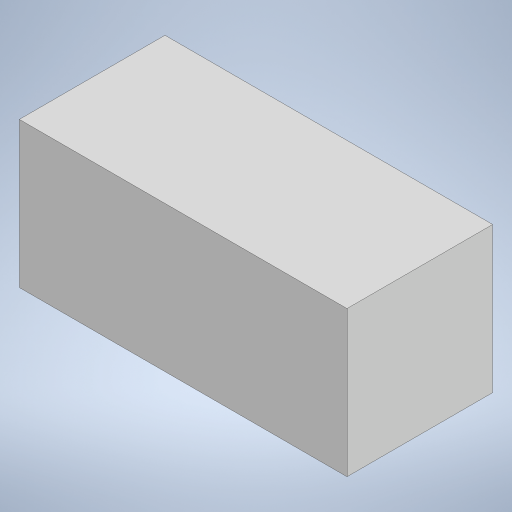
# Autodesk Inventor part: CinderBlock
Saved by Autodesk Inventor 2023 (Build 270158000, 158)
## iProperties
Created: 2022-09-11
Part Number: CinderBlock
Material: Generic
Document SubType Name: Modeling
Designer: PC
Density: 1 g/cm^3
Appearance: Default
Author: PC
Autodesk Inventor part; units mm, degrees
ref_plane "YZ Plane" through (0, 0, 0) normal (1, 0, 0) x (0, 1, 0)
ref_plane "XZ Plane" through (0, 0, 0) normal (0, 1, 0) x (-1, 0, 0)
ref_plane "XY Plane" through (0, 0, 0) normal (0, 0, 1) x (1, 0, 0)
sketch "Sketch1" plane through (0, 0, 0) normal (1, 0, 0) x (0, 1, 0)
  line L0 (0, 0) -> (203.2, 0)
  line L1 (203.2, 0) -> (203.2, -203.2)
  line L2 (203.2, -203.2) -> (0, -203.2)
  line L3 (0, -203.2) -> (0, 0)
  dimension "d0" = 203.2
  dimension "d1" = 203.2
  constraints: 8 end point, 2 parallel, 1 horizontal, 1 perpendicular
  measures "d0" distance of L1.end L2.end
  measures "d1" distance of L0.end L1.end
extrude "Extrusion1" add sketch "Sketch1" along normal blind 457.2
body "Solid1"
